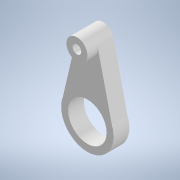
# Autodesk Inventor part: ClickSpringBacking
Saved by Autodesk Inventor 2022 (Build 260153000, 153)
## iProperties
Created: 2021-07-10
Part Number: ClickSpringBacking
Material: Generic
Document SubType Name: Modeling
Designer: teh18
Density: 1 g/cm^3
Appearance: Default
Mass: 6.16378 g
Surface Area: 33.0124 cm^2
Volume: 6.16378 cm^3
Author: teh18
Autodesk Inventor part; units mm, degrees
ref_plane "YZ Plane" through (0, 0, 0) normal (1, 0, 0) x (0, 1, 0)
ref_plane "XZ Plane" through (0, 0, 0) normal (0, 1, 0) x (-1, 0, 0)
ref_plane "XY Plane" through (0, 0, 0) normal (0, 0, 1) x (1, 0, 0)
sketch "Sketch1" plane through (0, 0, 0) normal (0, 0, 1) x (1, 0, 0)
  circle A0 centre (0, 0) radius 3.75 projected
  circle A1 centre (0, 0) radius 15 projected
  arc A2 (-0.5916, -14.9883) -> (-0.5916, -14.9883) centre (0, 0) ccw
  circle A3 centre (0, 38.847) radius 6
  circle A4 centre (0, 0) radius 11
  line L0 (5.8417, 40.216) -> (14.0107, 5.3571)
  line L1 (-14.0107, 5.3571) -> (-5.8417, 40.216)
  point P0 (-13.5955, 6.3373)
  point P1 (13.5955, 6.3373)
  point P2 (23.3721, 30.2282)
  dimension "d0" = 30
  dimension "d3" = 12
  dimension "d8" = 22
  dimension "d10" = 38.847
  constraints: 6 point on circle, 4 end point, 3 centre point, 2 tangent, 1 coincident, 1 vertical alignment
  measures "d0" diameter of A2
  measures "d3" diameter of A3
  measures "d8" diameter of A4
  measures "d10" distance of point (0, 0) A3.centre
extrude "Extrusion1" add sketch "Sketch1" along normal blind 9 contours A1 | A1 L1 A3 L0 | A3
sketch "Sketch2" plane through (0, 0, 9) normal (0, 0, 1) x (1, 0, 0)
  circle A0 centre (0, 38.847) radius 6
  arc A1 (5.8417, 40.216) -> (-5.8417, 40.216) centre (0, 38.847) ccw projected
  circle A2 centre (0, 38.847) radius 1.4
  point P0 (0, 0)
  dimension "d4" = 12
  dimension "d11" = 2.8
  constraints: 3 coincident, 2 centre point
  measures "d4" diameter of A0
  measures "d11" diameter of A2
extrude "Extrusion2" add sketch "Sketch2" along normal blind 6
sketch "Sketch3" plane through (0, 0, 0) normal (0, 0, -1) x (-1, 0, 0)
  arc A0 (5.8417, 40.216) -> (-5.8417, 40.216) centre (0, 38.847) ccw projected
  circle A1 centre (0, 38.847) radius 3
  point P0 (0, 0)
  dimension "d12" = 6
  constraints: 1 centre point, 1 coincident
  measures "d12" diameter of A1
extrude "Extrusion3" cut sketch "Sketch3" against normal blind 8
body "Solid1"
